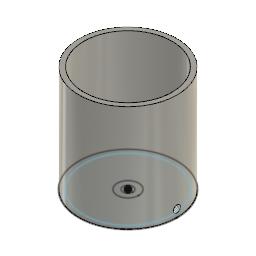
RUEDAS v0 (Autodesk Fusion 360 design; units mm, degrees)
Autodesk Fusion 360 part; units mm, degrees
sketch "Boceto1" plane through (0, 0, 0) normal (1, 0, 0) x (0, 1, 0)
sketch "Boceto2" plane through (0, 0, 0) normal (0, 0, 1) x (1, 0, 0)
  circle A0 centre (0, 0) radius 30
  circle A1 centre (0, 0) radius 3
  circle A2 centre (0, 0) radius 6.5
  line L0 (0, -30) -> (0.4326, -27.0314) construction
  circle A3 centre (0, 0) radius 27.0348
  dimension "d1" = 60
  dimension "d2" = 6
  dimension "d3" = 13
  dimension "d4" = 3
  constraint coincident A0.centre A1.centre
  constraint concentric A0 A1
  constraint coincident A0 L0.start
  constraint coincident L0.end A3
  measures "d1" diameter of A0
  measures "d2" diameter of A1
  measures "d3" diameter of A2
  measures "d4" distance of L0.start L0.end
extrude "Extruir1" add sketch "Boceto2" along normal blind 12 contours A2
extrude "Extruir3" add sketch "Boceto2" along normal blind 25 contours A3
extrude "Extruir4" add sketch "Boceto2" along normal blind 65 contours A0
hole "Agujero1" at (30, 0, 4.6114) direction (-1, 0, 0) diameter 4.234 depth 29 tip angle 180
thread "Rosca1" "ISO Metric profile 5.0 M5x0.8 6H"
extrude "Extruir2" [suppressed]
